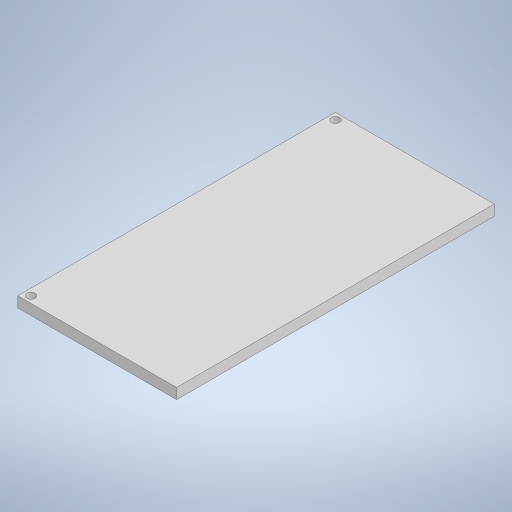
# Autodesk Inventor part: плата
Saved by Autodesk Inventor 2023.1 (Build 271208000, 208)
## iProperties
Created: 2026-02-22
Part Number: плата
Material: Типовые
Document SubType Name: Modeling
Designer: DELL
Density: 1 g/cm^3
Appearance: По умолчанию
Author: DELL
Autodesk Inventor part; units mm, degrees
ref_plane "YZ Plane" through (0, 0, 0) normal (1, 0, 0) x (0, 1, 0)
ref_plane "XZ Plane" through (0, 0, 0) normal (0, 1, 0) x (-1, 0, 0)
ref_plane "XY Plane" through (0, 0, 0) normal (0, 0, 1) x (1, 0, 0)
sketch "Эскиз1" plane through (0, 0, 0) normal (0, 1, 0) x (-1, 0, 0)
  line L0 (-30, -60) -> (30, -60)
  line L1 (30, -60) -> (30, 60)
  line L2 (30, 60) -> (-30, 60)
  line L3 (-30, 60) -> (-30, -60)
  line L4 (-30, -60) -> (30, 60) construction
  line L5 (30, -60) -> (-30, 60) construction
  point P0 (0, 0)
  dimension "d0" = 60
  dimension "d1" = 120
  constraints: 12 end point, 2 midpoint, 2 parallel, 1 horizontal, 1 perpendicular
  measures "d0" distance of L2.end L1.end
  measures "d1" distance of L1.end L0.end
extrude "Выдавливание1" add sketch "Эскиз1" along normal blind 4
sketch "Эскиз2" plane through (0, 4, 0) normal (0, 1, 0) x (1, 0, 0)
  line L0 (-27.5, -57.5) -> (-27.5, 57.5) construction
  line L1 (30, -60) -> (30, 60) projected
  line L2 (30, 0) -> (-30, 0) construction
  line L3 (-30, 60) -> (-30, -60) projected
  circle A0 centre (-27.5, -57.5) radius 1.6
  circle A1 centre (-27.5, 57.5) radius 1.6
  point P0 (0, 0)
  point P1 (-27.5, 0)
  dimension "d4" = 115
  dimension "d5" = 3.2
  dimension "d6" = 3.2
  dimension "d7" = 2.5
  constraints: 4 end point, 3 midpoint, 2 centre point, 2 coincident, 1 point on line, 1 vertical
  measures "d4" distance of L0.start L0.end
  measures "d5" diameter of A0
  measures "d6" diameter of A1
  measures "d7" distance from line of L3 A1.centre
extrude "Выдавливание2" cut sketch "Эскиз2" against normal blind 4
